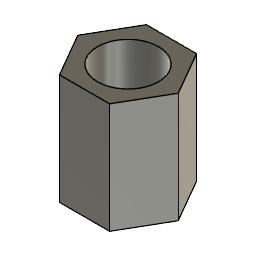
1in Offset (Autodesk Fusion 360 design; units mm, degrees)
Autodesk Fusion 360 part; units mm, degrees
sketch "Sketch1" plane through (0, 0, 0) normal (0, 0, 1) x (1, 0, 0)
  line L0 (-5.7735, 10) -> (-11.547, 0)
  line L1 (-11.547, 0) -> (-5.7735, -10)
  line L2 (-5.7735, -10) -> (5.7735, -10)
  line L3 (5.7735, -10) -> (11.547, 0)
  line L4 (11.547, 0) -> (5.7735, 10)
  line L5 (5.7735, 10) -> (-5.7735, 10)
  circle A0 centre (0, 0) radius 7
  dimension "d1" = 10
  constraint coincident A0.centre origin
  measures "d1" distance of A0.centre L5
extrude "Extrude1" add sketch "Sketch1" along normal blind 25.4
